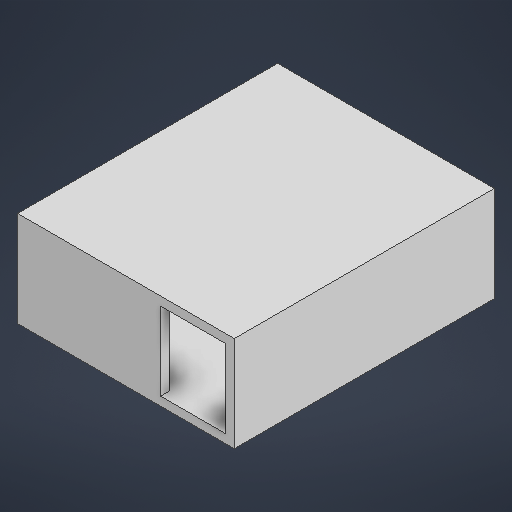
# Autodesk Inventor part: Schutzbox technik
Saved by Autodesk Inventor 2026.2 (Build 302298000, 298)
## iProperties
Created: 2026-01-21
Part Number: Schutzbox technik
Material: Generisch
Document SubType Name: Modeling
Designer: Schally
Density: 1 g/cm^3
Appearance: Vorgabe
Author: Schally
Autodesk Inventor part; units mm, degrees
ref_plane "YZ Plane" through (0, 0, 0) normal (1, 0, 0) x (0, 1, 0)
ref_plane "XZ Plane" through (0, 0, 0) normal (0, 1, 0) x (-1, 0, 0)
ref_plane "XY Plane" through (0, 0, 0) normal (0, 0, 1) x (1, 0, 0)
sketch "Skizze1" plane through (0, 0, 0) normal (0, 1, 0) x (-1, 0, 0)
  line L0 (0, 0) -> (-100, 0)
  line L1 (-100, 0) -> (-100, -120)
  line L2 (-100, -120) -> (0, -120)
  line L3 (0, -120) -> (0, 0)
  dimension "d0" = 100
  dimension "d1" = 120
  constraints: 8 end point, 2 parallel, 1 horizontal, 1 perpendicular
  measures "d0" distance between parallel lines of L3 L1
  measures "d1" distance between parallel lines of L0 L2
extrude "Extrusion1" add sketch "Skizze1" along normal blind 4
sketch "Skizze2" plane through (0, 0, 0) normal (0, -1, 0) x (1, 0, 0)
  line L0 (100, 0) -> (100, -120) projected
  line L1 (100, -120) -> (0, -120) projected
  line L2 (0, -120) -> (0, 0) projected
  line L3 (0, 0) -> (100, 0) projected
  line L4 (4, -116) -> (96, -116)
  line L5 (96, -116) -> (96, -4)
  line L6 (96, -4) -> (4, -4)
  line L7 (4, -4) -> (4, -116)
  line L8 (4, -116) -> (4, -120)
  line L9 (96, -116) -> (96, -120)
  dimension "d4" = 4
  constraints: 12 end point, 2 perpendicular, 2 point on line, 3 other
  measures "d4" distance between parallel lines of L1 L4
extrude "Extrusion2" add sketch "Skizze2" against normal blind 40 contours L0 L1 L9 L5 L6 L7 L8 L2 L3
sketch "Skizze3" plane through (0, 40, 0) normal (0, 1, 0) x (1, 0, 0)
  line L0 (100, 120) -> (0, 120) projected
  line L1 (100, 0) -> (100, 120) projected
  line L2 (0, 0) -> (100, 0) projected
  line L3 (0, 120) -> (0, 0) projected
extrude "Extrusion3" add sketch "Skizze3" along normal blind 4
sketch "Skizze4" plane through (0, 0, 0) normal (0, 0, 1) x (1, 0, 0)
  line L0 (4, 4) -> (96, 4) construction
  line L1 (4, 4) -> (4, 40) construction
  line L2 (96, 40) -> (4, 40) construction
  line L3 (96, 4) -> (96, 40) construction
  line L4 (96, 40) -> (66, 40)
  line L5 (66, 40) -> (66, 4)
  line L6 (66, 4) -> (96, 4)
  line L7 (96, 4) -> (96, 40)
  point P0 (0, 0)
  dimension "d9" = 30
  constraints: 8 end point, 2 parallel, 1 horizontal, 1 perpendicular, 1 point on line
  measures "d9" distance of L6.end L5.end
extrude "Extrusion4" cut sketch "Skizze4" against normal blind 4
